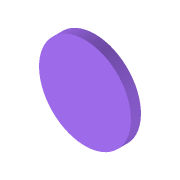
# Autodesk Inventor part: 50_ETL_Membrane_Mould_Upper_v0
Saved by Autodesk Inventor 2022 (Build 260153000, 153)
## iProperties
Created: 2021-12-31
Part Number: 50_ETL_Membrane_Mould_Upper_v0
Material: Generisch
Document SubType Name: Modeling
Designer: diederichbenedict
Density: 1 g/cm^3
Appearance: Violett
Author: diederichbenedict
Autodesk Inventor part; units mm, degrees
ref_plane "YZ Plane" through (0, 0, 0) normal (1, 0, 0) x (0, 1, 0)
ref_plane "XZ Plane" through (0, 0, 0) normal (0, 1, 0) x (-1, 0, 0)
ref_plane "XY Plane" through (0, 0, 0) normal (0, 0, 1) x (1, 0, 0)
sketch "Skizze1" plane through (0, 0, 0) normal (1, 0, 0) x (0, 1, 0)
  line L0 (5, 0) -> (-30, 0) projected
  line L1 (5, -3) -> (5, 0)
  line L2 (-3.9492, 2.2) -> (-21.0508, 2.2) projected
  line L3 (-6.3, 0.7) -> (-18.7, 0.7) projected
  line L4 (-12.5, 0.7) -> (-12.5, 5.3428)
  line L5 (5, 0) -> (-2.1515, 0)
  line L6 (-18.5, 0.7) -> (-6.5, 0.7) construction
  line L7 (-6.5, 0.7) -> (-6.5, 0.9) construction
  line L8 (-6.5, 0.9) -> (-18.5, 0.9) construction
  line L9 (-18.5, 0.9) -> (-18.5, 0.7) construction
  line L10 (-18.5, 0.7) -> (-6.5, 0.9) construction
  line L11 (-6.5, 0.7) -> (-18.5, 0.9) construction
  line L12 (-6.3, 0.7) -> (-7.4658, 0.7) construction
  line L13 (-12.5, 0.9) -> (-6.4, 0.9)
  line L14 (-6.4, 0.9) -> (-6.4, 0.7)
  line L15 (-6.3, 0.7) -> (-6.4, 0.7)
  line L16 (-12.5, 0.9) -> (-12.5, 3.9)
  line L17 (-12.5, 3.9) -> (5, 3.9)
  line L18 (5, 3.9) -> (5, 0)
  line L19 (-4.8, 2.2) -> (-6.3, 0.7)
  line L20 (-3.9492, 2.2) -> (-21.0508, 2.2) projected
  line L21 (-1.7515, 0) -> (-3.9503, 2.1989)
  line L22 (-5.7431, 0.4) -> (-4.5431, 1.6) construction
  line L23 (-4.1977, 1.6) -> (-20.8023, 1.6) construction
  line L24 (-4.1977, 1.6) -> (-3.1977, 0.6) construction
  line L25 (-4.1977, 1.6) -> (-20.8023, 1.6) construction
  line L26 (5, 3.9) -> (7.4806, 3.9)
  line L27 (7.4806, 3.9) -> (7.4806, -1.0263)
  line L28 (7.4806, -1.0263) -> (5.458, -1.0263)
  line L29 (5, 0) -> (5.2, 0)
  line L30 (5.2, 0) -> (5.4633, -1.0263)
  point P0 (0, 0)
  point P1 (-5.8, 2.2)
  point P2 (-12.5, 0.8)
  point P3 (-12.5, 0.9)
  point P4 (-1.7515, 0)
  dimension "d0" = 12
  dimension "d1" = 0.2
  dimension "d2" = 6.1
  dimension "d3" = 3
  dimension "d5" = 0.2
  constraints: 50 end point, 7 perpendicular, 7 point on line, 5 midpoint, 2 horizontal, 2 parallel, 2 vertical, 14 other
  measures "d0" distance of L8.end L7.end
  measures "d1" distance of L7.end L6.end
  measures "d2" distance of L13.start L13.end
  measures "d3" distance of L13.start L16.end
  measures "d5" distance of L0.start L29.end
revolve "Umdrehung1" add sketch "Skizze1" angle 360 about axis through (0, -12.5, 0.7) along (0, 0, 1) contours L0 L21 L2 L4 L17 L18 | L18 L26 L27 L28 L30 L29 | L19 L3 L14 L13 L4 L2
